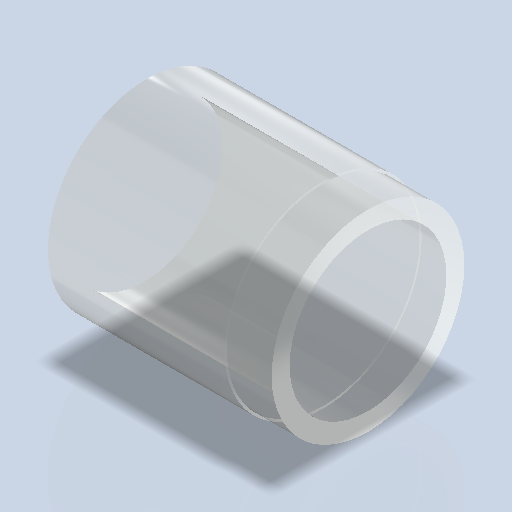
# Autodesk Inventor part: Zylinder_laufbuechse
Saved by Autodesk Inventor 2024 (Build 280153000, 153)
## iProperties
Created: 2024-02-29
Part Number: Zylinder_laufbuechse
Material: Glas
Document SubType Name: Modeling
Designer: ffogue
Density: 2.18 g/cm^3
Appearance: Klar
Author: ffogue
Autodesk Inventor part; units mm, degrees
ref_plane "YZ Plane" through (0, 0, 0) normal (1, 0, 0) x (0, 1, 0)
ref_plane "XZ Plane" through (0, 0, 0) normal (0, 1, 0) x (-1, 0, 0)
ref_plane "XY Plane" through (0, 0, 0) normal (0, 0, 1) x (1, 0, 0)
sketch "Skizze1" plane through (0, 0, 0) normal (0, 0, 1) x (1, 0, 0)
  line L0 (0, 0) -> (0, 22)
  line L1 (0, 22) -> (40, 22)
  line L2 (40, 22) -> (40, 21.5)
  line L3 (40, 21.5) -> (50, 21.5)
  line L4 (50, 21.5) -> (50, 0)
  line L5 (50, 0) -> (0, 0)
  dimension "d0" = 44
  dimension "d1" = 43
  dimension "d2" = 40
  dimension "d3" = 50
  constraints: 12 end point, 5 perpendicular, 1 vertical
  measures "d0" diameter of L1 L5
  measures "d1" diameter of L3 L5
  measures "d2" distance between parallel lines of L2 L0
  measures "d3" distance between parallel lines of L4 L0
revolve "Umdrehung1" add sketch "Skizze1" angle 360 about axis through (50, 0, 0) along (-1, 0, 0)
chamfer "Fasen1" distance 2 angle 15 1 edges at (0, -22, 0) measured on face at (0, -5.3524, -1.755)
sketch "Skizze2" plane through (50, 0, 0) normal (1, 0, 0) x (0, 0, -1)
  circle A0 centre (0, 0) radius 17.5
  dimension "d8" = 35
  constraints: 1 centre point, 1 coincident
  measures "d8" diameter of A0
extrude "Extrusion1" cut sketch "Skizze2" against normal up to surface (50 mm away)
